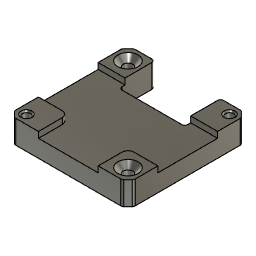
mount v1 (Autodesk Fusion 360 design; units mm, degrees)
Autodesk Fusion 360 part; units mm, degrees
note: some values were not read from the file. Set by a fixed rule: which sketch regions a step uses.
sketch "Sketch1" plane through (0, 0, 0) normal (0, 0, 1) x (1, 0, 0)
  line L0 (20, 20) -> (-20, 20)
  line L1 (-20, 20) -> (-20, -20)
  line L2 (-20, -20) -> (20, -20)
  line L3 (20, -20) -> (20, 20)
  line L4 (20, 20) -> (-20, -20) construction
  line L5 (-20, 20) -> (20, -20) construction
  dimension "d1" = 40
  dimension "d2" = 40
  constraint horizontal L0
  constraint perpendicular L0 L1
  constraint parallel L0 L2
  constraint parallel L1 L3
  constraint coincident L4 origin
  constraint coincident L5 origin
  measures "d1" distance of L1.end L2.end
  measures "d2" distance of L0.end L1.end
extrude "Extrude1" add sketch "Sketch1" along normal blind 8
sketch "Sketch2" plane through (0, 0, 8) normal (0, 0, 1) x (-1, 0, 0)
  line L0 (-20, 20) -> (-20, -20)
  line L1 (-20, -20) -> (20, -20)
  line L2 (20, -20) -> (20, 20)
  line L3 (20, 20) -> (-20, 20)
  circle A0 centre (15.5, -15.5) radius 1.6
  line L4 (-15.5, -15.5) -> (15.5, -15.5) construction
  line L5 (15.5, -15.5) -> (15.5, 15.5) construction
  line L6 (15.5, 15.5) -> (-15.5, 15.5) construction
  line L7 (-15.5, 15.5) -> (-15.5, -15.5) construction
  line L8 (-15.5, -15.5) -> (15.5, 15.5) construction
  line L9 (15.5, -15.5) -> (-15.5, 15.5) construction
  circle A1 centre (-15.5, 15.5) radius 1.6
  dimension "d5" = 3.2
  dimension "d6" = 31
  dimension "d7" = 31
  dimension "d8" = 3.2
  constraint horizontal L4
  constraint perpendicular L4 L5
  constraint parallel L4 L6
  constraint parallel L5 L7
  constraint coincident L8 origin
  constraint coincident L9 origin
  constraint coincident A0.centre L4.end
  constraint coincident L6.end L7.start
  measures "d5" diameter of A0
  measures "d6" distance of L4.start A0.centre
  measures "d7" distance of L4.start L6.end
  measures "d8" diameter of A1
extrude "Extrude2" cut sketch "Sketch2" against normal blind 15 contours A0 | A1
sketch "Sketch3" plane through (0, 0, 8) normal (0, 0, 1) x (-1, 0, 0)
  circle A0 centre (15.5, -15.5) radius 1.6
  circle A1 centre (-15.5, 15.5) radius 1.6
  line L0 (-20, 20) -> (-20, -20)
  line L1 (-20, -20) -> (20, -20)
  line L2 (20, -20) -> (20, 20)
  line L3 (20, 20) -> (-20, 20)
  line L4 (-17, -17) -> (17, -17) construction
  line L5 (17, -17) -> (17, 17) construction
  line L6 (17, 17) -> (-17, 17) construction
  line L7 (-17, 17) -> (-17, -17) construction
  line L8 (-17, -17) -> (17, 17) construction
  line L9 (17, -17) -> (-17, 17) construction
  circle A2 centre (-17, -17) radius 1.35
  circle A3 centre (17, 17) radius 1.35
  dimension "d11" = 34
  dimension "d12" = 34
  dimension "d13" = 2.7
  dimension "d14" = 2.7
  constraint horizontal L4
  constraint perpendicular L4 L5
  constraint parallel L4 L6
  constraint parallel L5 L7
  constraint coincident L8 origin
  constraint coincident L9 origin
  constraint coincident L4.start L7.end
  constraint coincident L5.end L6.start
  measures "d11" distance of L5.end L6.end
  measures "d12" distance of L4.end L5.end
  measures "d13" diameter of A2
  measures "d14" diameter of A3
extrude "Extrude3" cut sketch "Sketch3" against normal blind 12 contours A2 | A3
chamfer "Chamfer1" distance 1.8 angle 45 2 edges at (-14.0083, 14.9214, 8) (16.9917, -16.0786, 8)
chamfer "Chamfer2" distance 2 angle 45 4 edges at (20, -20, 4) (-20, -20, 4) (20, 20, 4) (-20, 20, 4)
sketch "Sketch4" plane through (0, 0, 8) normal (0, 0, 1) x (-1, 0, 0)
  circle A0 centre (15.5, -15.5) radius 3.4
  circle A1 centre (-17, -17) radius 1.35
  circle A2 centre (17, 17) radius 1.35
  line L0 (18, -20) -> (20, -18)
  line L1 (20, -18) -> (20, 18)
  line L2 (20, 18) -> (18, 20)
  line L3 (18, 20) -> (-18, 20)
  line L4 (-18, 20) -> (-20, 18)
  line L5 (-20, 18) -> (-20, -18)
  line L6 (-20, -18) -> (-18, -20)
  line L7 (-18, -20) -> (18, -20)
  circle A3 centre (-15.5, 15.5) radius 3.4
chamfer "Chamfer3" distance 0.5 angle 45 2 edges at (-15.7414, -17.4882, 8) (18.2586, 16.5118, 8)
sketch "Sketch5" plane through (0, 0, 8) normal (0, 0, 1) x (-1, 0, 0)
  line L0 (11, -20) -> (-11, -20)
  line L1 (-11, -20) -> (-11, -8)
  line L2 (-11, -8) -> (11, -8)
  line L3 (11, -8) -> (11, -20)
  line L4 (-18, -20) -> (18, -20)
  point P0 (0, -8)
  dimension "d20" = 22
  dimension "d21" = 12
  constraint horizontal L0
  constraint vertical L1
  constraint horizontal L2
  constraint vertical L3
  constraint midpoint L2 P0
  constraint vertical P0 origin
  constraint coincident L0.end L4
  measures "d20" distance of L1.end L2.end
  measures "d21" distance of L0.end L1.end
extrude "Extrude4" cut sketch "Sketch5" against normal blind 15
fillet "Fillet1" radius 1 4 edges at (-11, 8, 4) (11, 8, 4) (11, 20, 4) (-11, 20, 4)
fillet "Fillet1" radius 1 8 edges at (-18, 20, 4) (-20, 18, 4) (-20, -18, 4) (-18, -20, 4) (18, -20, 4) (20, -18, 4) (20, 18, 4) (18, 20, 4)
chamfer "Chamfer4" distance 0.2 angle 45 1 faces at (-3.942, -7.6818, 0)
sketch "Sketch6" plane through (0, 0, 8) normal (0, 0, 1) x (-1, 0, 0)
  circle A0 centre (17, 17) radius 1.85
  circle A1 centre (15.5, -15.5) radius 3.4
  circle A2 centre (-15.5, 15.5) radius 3.4
  circle A3 centre (-17, -17) radius 1.85
  arc A4 (-18.2929, -19.7071) -> (-17.5858, -20) centre (-17.5858, -19) ccw
  line L0 (-17.5858, -20) -> (-12, -20)
  arc A5 (-12, -20) -> (-11, -19) centre (-12, -19) ccw
  line L1 (-11, -19) -> (-11, -9)
  arc A6 (-10, -8) -> (-11, -9) centre (-10, -9) ccw
  line L2 (-10, -8) -> (10, -8)
  arc A7 (11, -9) -> (10, -8) centre (10, -9) ccw
  line L3 (11, -9) -> (11, -19)
  arc A8 (11, -19) -> (12, -20) centre (12, -19) ccw
  line L4 (12, -20) -> (17.5858, -20)
  arc A9 (17.5858, -20) -> (18.2929, -19.7071) centre (17.5858, -19) ccw
  line L5 (18.2929, -19.7071) -> (19.7071, -18.2929)
  arc A10 (19.7071, -18.2929) -> (20, -17.5858) centre (19, -17.5858) ccw
  line L6 (20, -17.5858) -> (20, 17.5858)
  arc A11 (20, 17.5858) -> (19.7071, 18.2929) centre (19, 17.5858) ccw
  line L7 (19.7071, 18.2929) -> (18.2929, 19.7071)
  arc A12 (18.2929, 19.7071) -> (17.5858, 20) centre (17.5858, 19) ccw
  line L8 (17.5858, 20) -> (-17.5858, 20)
  arc A13 (-17.5858, 20) -> (-18.2929, 19.7071) centre (-17.5858, 19) ccw
  line L9 (-18.2929, 19.7071) -> (-19.7071, 18.2929)
  arc A14 (-19.7071, 18.2929) -> (-20, 17.5858) centre (-19, 17.5858) ccw
  line L10 (-20, 17.5858) -> (-20, -17.5858)
  arc A15 (-20, -17.5858) -> (-19.7071, -18.2929) centre (-19, -17.5858) ccw
  line L11 (-19.7071, -18.2929) -> (-18.2929, -19.7071)
  line L12 (-10, 20) -> (-10, 10)
  line L13 (-10, 10) -> (-20, 10)
  line L14 (-20, -10) -> (-11, -10)
  line L15 (0, -2.5) -> (0, -20)
  line L16 (10, 20) -> (10, 10)
  line L17 (10, 10) -> (20, 10)
  line L18 (20, -10) -> (11, -10)
  line L19 (11, -10) -> (10.0078, -10.7171)
  dimension "d29" = 10
  dimension "d32" = 10
  dimension "d37" = 10
  constraint coincident L8 L12.start
  constraint perpendicular L8 L12
  constraint coincident L10 L13.end
  constraint perpendicular L10 L13
  constraint coincident L10 L14.start
  constraint perpendicular L10 L14
  constraint symmetric L12.start L15 L16.start
  constraint symmetric L12.end L15 L16.end
  constraint symmetric L13.end L15 L17.end
  constraint symmetric L14.start L15 L18.start
  constraint symmetric L14.end L15 L18.end
  constraint coincident L1 L14.end
  measures "d29" distance of L10 L12
  measures "d32" distance of L8 L13
  measures "d37" distance of L0 L14
extrude "Extrude5" cut sketch "Sketch6" against normal blind 2 contours L1 A6 L2 A7 L3 L6 L8 L10 L12 L13 L14 L16 L17 L18
fillet "Fillet2" radius 2 2 edges at (10, -10, 7) (-10, -10, 7)
